Autodesk Fusion 360 part; units mm, degrees
(part 3 of 3)
equation "d13 = 1.525 mm + 0.5 mm"
named bodies: "PCB Motherboard", "Connection", "Top Layer", "Bottom Layer", "Connection (1)", "Connection (2)", "Connection (3)", "Connection (4)", "Connection (5)", "Connection (6)", "Connection (7)", "Connection (8)", "Connection (9)", "Connection (10)", "Connection (11)", "Connection (12)", "Connection (13)", "Connection (14)", "Top Layer (1)", "Top Layer (2)", "Top Layer (3)", "Top Layer (4)", "Top Layer (5)", "Top Layer (6)", "Top Layer (7)", "Top Layer (8)", "Top Layer (9)", "Top Layer (10)", "Top Layer (11)", "Top Layer (12)", "Top Layer (13)", "Top Layer (14)", "Bottom Layer (1)", "Bottom Layer (2)", "Bottom Layer (3)", "Bottom Layer (4)", "Bottom Layer (5)", "Bottom Layer (6)", "Bottom Layer (7)", "Bottom Layer (8)", "Bottom Layer (9)", "Bottom Layer (10)", "Bottom Layer (11)", "Bottom Layer (12)", "Bottom Layer (13)", "Bottom Layer (14)", "Connection (15)", "Connection (16)", "Connection (17)", "Connection (18)", "Connection (19)", "Connection (20)", "Connection (21)", "Connection (22)", "Connection (23)", "Connection (24)", "Connection (25)", "Connection (26)", "Connection (27)", "Connection (28)", "Connection (29)", "Connection (30)", "Connection (31)", "Connection (32)", "Connection (33)", "Connection (34)", "Connection (35)", "Connection (36)", "Connection (37)", "Connection (38)", "Connection (39)", "Connection (40)", "Connection (41)", "Connection (42)", "Connection (43)", "Connection (44)", "Connection (45)", "Connection (46)", "Connection (47)", "Connection (48)", "Connection (49)", "Connection (50)", "Connection (51)", "Connection (52)", "Connection (53)", "Connection (54)", "Connection (55)", "Connection (56)", "Connection (57)", "Connection (58)", "Connection (59)", "Connection (60)", "Connection (61)", "Connection (62)", "Connection (63)", "Connection (64)", "Connection (65)", "Connection (66)", "Connection (67)", "Connection (68)", "Connection (69)", "Connection (70)", "Connection (71)", "Connection (72)", "Connection (73)", "Connection (74)", "Connection (75)", "Connection (76)", "Connection (77)", "Connection (78)", "Connection (79)", "Connection (80)", "Connection (81)", "Connection (82)", "Connection (83)", "Connection (84)", "Connection (85)", "Connection (86)", "Connection (87)", "Connection (88)", "Connection (89)", "Connection (90)", "Connection (91)", "Connection (92)", "Connection (93)", "Connection (94)", "Connection (95)", "Connection (96)", "Connection (97)", "Connection (98)", "Connection (99)", "Connection (100)", "Connection (101)", "Connection (102)", "Connection (103)", "Connection (104)", "Connection (105)", "Connection (106)", "Connection (107)", "Connection (108)", "Connection (109)", "Connection (110)", "Connection (111)", "Connection (112)", "Connection (113)", "Connection (114)", "Connection (115)", "Connection (116)", "Connection (117)", "Connection (118)", "Connection (119)", "Connection (120)", "Connection (121)", "Connection (122)", "Connection (123)", "Connection (124)", "Connection (125)", "Connection (126)", "Connection (127)", "Connection (128)", "Connection (129)", "Connection (130)", "Connection (131)", "Connection (132)", "Connection (133)", "Connection (134)", "Connection (135)", "Connection (136)", "Connection (137)", "Connection (138)", "Connection (139)", "Connection (140)", "Connection (141)", "Connection (142)", "Connection (143)", "Connection (144)", "Connection (145)", "Connection (146)", "Connection (147)", "Connection (148)", "Connection (149)", "Connection (150)", "Connection (151)", "Connection (152)", "Connection (153)", "Connection (154)", "Connection (155)", "Connection (156)", "Connection (157)", "Connection (158)", "Connection (159)", "Connection (160)", "Connection (161)", "Connection (162)", "Connection (163)", "Connection (164)", "Connection (165)", "Connection (166)", "Connection (167)", "Connection (168)", "Connection (169)", "Connection (170)", "Connection (171)", "Connection (172)", "Connection (173)", "Connection (174)", "Connection (175)", "Connection (176)", "Connection (177)", "Connection (178)", "Connection (179)", "Connection (180)", "Connection (181)", "Connection (182)", "Connection (183)", "Connection (184)", "Connection (185)", "Connection (186)", "Connection (187)", "Connection (188)", "Connection (189)", "Connection (190)", "Connection (191)", "Connection (192)", "Connection (193)", "Connection (194)", "Connection (195)", "Connection (196)", "Connection (197)", "Connection (198)", "Connection (199)", "Connection (200)", "Connection (201)", "Connection (202)", "Connection (203)", "Connection (204)", "Connection (205)", "Connection (206)", "Connection (207)", "Connection (208)", "Connection (209)", "Connection (210)", "Connection (211)", "Connection (212)", "Connection (213)", "Connection (214)", "Connection (215)", "Connection (216)", "Connection (217)", "Connection (218)", "Connection (219)", "Connection (220)", "Connection (221)", "Connection (222)", "Connection (223)", "Connection (224)", "Connection (225)", "Connection (226)", "Connection (227)", "Connection (228)", "Connection (229)", "Connection (230)", "Connection (231)", "Connection (232)", "Connection (233)", "Connection (234)", "Connection (235)", "Connection (236)", "Connection (237)", "Connection (238)", "Connection (239)", "Connection (240)", "Connection (241)", "Connection (242)", "Connection (243)", "Connection (244)", "Connection (245)", "Connection (246)", "Connection (247)", "Connection (248)", "Connection (249)", "Connection (250)", "Connection (251)", "Connection (252)", "Connection (253)", "Connection (254)", "Connection (255)", "Connection (256)", "Connection (257)", "Connection (258)", "Connection (259)", "Connection (260)", "Connection (261)", "Connection (262)", "Connection (263)", "Connection (264)", "Connection (265)", "Connection (266)", "Connection (267)", "Connection (268)", "Connection (269)", "Connection (270)", "Connection (271)", "Connection (272)", "Connection (273)", "Connection (274)", "Connection (275)", "Connection (276)", "Connection (277)", "Connection (278)", "Connection (279)", "Connection (280)", "Connection (281)", "Connection (282)", "Connection (283)", "Connection (284)", "Connection (285)", "Connection (286)", "Connection (287)", "Connection (288)", "Connection (289)", "Connection (290)", "Connection (291)", "Connection (292)", "Connection (293)", "Connection (294)", "Connection (295)", "Connection (296)", "Connection (297)", "Connection (298)", "Connection (299)", "Connection (300)", "Connection (301)", "Connection (302)", "Connection (303)", "Connection (304)", "Connection (305)", "Connection (306)", "Connection (307)", "Connection (308)", "Connection (309)", "Connection (310)", "Connection (311)", "Connection (312)", "Connection (313)", "Connection (314)", "Connection (315)", "Connection (316)", "Connection (317)", "Connection (318)", "Connection (319)", "Connection (320)", "Connection (321)", "Connection (322)", "Connection (323)", "Connection (324)", "Connection (325)", "Connection (326)", "Connection (327)", "Connection (328)", "Connection (329)", "Connection (330)", "Connection (331)", "Connection (332)", "Connection (333)", "Connection (334)", "Connection (335)", "Connection (336)", "Connection (337)", "Connection (338)", "Connection (339)", "Connection (340)", "Connection (341)", "Connection (342)", "Connection (343)", "Connection (344)", "Connection (345)", "Connection (346)", "Connection (347)", "Connection (348)", "Connection (349)", "Connection (350)", "Connection (351)", "Connection (352)", "Connection (353)", "Connection (354)", "Connection (355)", "Connection (356)", "Connection (357)", "Connection (358)", "Connection (359)", "Connection (360)", "Connection (361)", "Connection (362)", "Connection (363)", "Connection (364)", "Connection (365)", "Connection (366)", "Connection (367)", "Connection (368)", "Connection (369)", "Connection (370)", "Connection (371)", "Connection (372)", "Connection (373)", "Connection (374)", "Top Layer (15)", "Top Layer (16)", "Top Layer (17)", "Top Layer (18)", "Top Layer (19)", "Top Layer (20)", "Top Layer (21)", "Top Layer (22)", "Top Layer (23)", "Top Layer (24)", "Top Layer (25)", "Top Layer (26)", "Top Layer (27)", "Top Layer (28)", "Top Layer (29)", "Top Layer (30)", "Top Layer (31)", "Top Layer (32)", "Top Layer (33)", "Top Layer (34)", "Top Layer (35)", "Top Layer (36)", "Top Layer (37)", "Top Layer (38)", "Top Layer (39)", "Top Layer (40)", "Top Layer (41)", "Top Layer (42)", "Top Layer (43)", "Top Layer (44)", "Top Layer (45)", "Top Layer (46)", "Top Layer (47)", "Top Layer (48)", "Top Layer (49)", "Top Layer (50)", "Top Layer (51)", "Top Layer (52)", "Top Layer (53)", "Top Layer (54)", "Top Layer (55)", "Top Layer (56)", "Top Layer (57)", "Top Layer (58)", "Top Layer (59)", "Top Layer (60)", "Top Layer (61)", "Top Layer (62)", "Top Layer (63)", "Top Layer (64)", "Top Layer (65)", "Top Layer (66)", "Top Layer (67)", "Top Layer (68)", "Top Layer (69)", "Top Layer (70)", "Top Layer (71)", "Top Layer (72)", "Top Layer (73)", "Top Layer (74)", "Top Layer (75)", "Top Layer (76)", "Top Layer (77)", "Top Layer (78)", "Top Layer (79)", "Top Layer (80)", "Top Layer (81)", "Top Layer (82)", "Top Layer (83)", "Top Layer (84)", "Top Layer (85)", "Top Layer (86)", "Top Layer (87)", "Top Layer (88)", "Top Layer (89)", "Top Layer (90)", "Top Layer (91)", "Top Layer (92)", "Top Layer (93)", "Top Layer (94)", "Top Layer (95)", "Top Layer (96)", "Top Layer (97)", "Top Layer (98)", "Top Layer (99)", "Top Layer (100)", "Top Layer (101)", "Top Layer (102)", "Top Layer (103)", "Top Layer (104)", "Top Layer (105)", "Top Layer (106)", "Top Layer (107)", "Top Layer (108)", "Top Layer (109)", "Top Layer (110)", "Top Layer (111)", "Top Layer (112)", "Top Layer (113)", "Top Layer (114)", "Top Layer (115)", "Top Layer (116)", "Top Layer (117)", "Top Layer (118)", "Top Layer (119)", "Top Layer (120)", "Top Layer (121)", "Top Layer (122)", "Top Layer (123)", "Top Layer (124)", "Top Layer (125)", "Top Layer (126)", "Top Layer (127)", "Top Layer (128)", "Top Layer (129)", "Top Layer (130)", "Top Layer (131)", "Top Layer (132)", "Top Layer (133)", "Top Layer (134)", "Top Layer (135)", "Top Layer (136)", "Top Layer (137)", "Top Layer (138)", "Top Layer (139)", "Top Layer (140)", "Top Layer (141)", "Top Layer (142)", "Top Layer (143)", "Top Layer (144)", "Top Layer (145)", "Top Layer (146)", "Top Layer (147)", "Top Layer (148)", "Top Layer (149)", "Top Layer (150)", "Top Layer (151)", "Top Layer (152)", "Top Layer (153)", "Top Layer (154)", "Top Layer (155)", "Top Layer (156)", "Top Layer (157)", "Top Layer (158)", "Top Layer (159)", "Top Layer (160)", "Top Layer (161)", "Top Layer (162)", "Top Layer (163)", "Top Layer (164)", "Top Layer (165)", "Top Layer (166)", "Top Layer (167)", "Top Layer (168)", "Top Layer (169)", "Top Layer (170)", "Top Layer (171)", "Top Layer (172)", "Top Layer (173)", "Top Layer (174)", "Top Layer (175)", "Top Layer (176)", "Top Layer (177)", "Top Layer (178)", "Top Layer (179)", "Top Layer (180)", "Top Layer (181)", "Top Layer (182)", "Top Layer (183)", "Top Layer (184)", "Top Layer (185)", "Top Layer (186)", "Top Layer (187)", "Top Layer (188)", "Top Layer (189)", "Top Layer (190)", "Top Layer (191)", "Top Layer (192)", "Top Layer (193)", "Top Layer (194)", "Top Layer (195)", "Top Layer (196)", "Top Layer (197)", "Top Layer (198)", "Top Layer (199)", "Top Layer (200)", "Top Layer (201)", "Top Layer (202)", "Top Layer (203)", "Top Layer (204)", "Top Layer (205)", "Top Layer (206)", "Top Layer (207)", "Top Layer (208)", "Top Layer (209)", "Top Layer (210)", "Top Layer (211)", "Top Layer (212)", "Top Layer (213)", "Top Layer (214)", "Top Layer (215)", "Top Layer (216)", "Top Layer (217)", "Top Layer (218)", "Top Layer (219)", "Top Layer (220)", "Top Layer (221)", "Top Layer (222)", "Top Layer (223)", "Top Layer (224)", "Top Layer (225)", "Top Layer (226)", "Top Layer (227)", "Top Layer (228)", "Top Layer (229)", "Top Layer (230)", "Top Layer (231)", "Top Layer (232)", "Top Layer (233)", "Top Layer (234)", "Top Layer (235)", "Top Layer (236)", "Top Layer (237)", "Top Layer (238)", "Top Layer (239)", "Top Layer (240)", "Top Layer (241)", "Top Layer (242)", "Top Layer (243)", "Top Layer (244)", "Top Layer (245)", "Top Layer (246)", "Top Layer (247)", "Top Layer (248)", "Top Layer (249)", "Top Layer (250)", "Top Layer (251)", "Top Layer (252)", "Top Layer (253)", "Top Layer (254)", "Top Layer (255)", "Top Layer (256)", "Top Layer (257)", "Top Layer (258)", "Top Layer (259)", "Top Layer (260)", "Top Layer (261)", "Top Layer (262)", "Top Layer (263)", "Top Layer (264)", "Top Layer (265)", "Top Layer (266)", "Top Layer (267)", "Top Layer (268)", "Top Layer (269)", "Top Layer (270)", "Top Layer (271)", "Top Layer (272)", "Top Layer (273)", "Top Layer (274)", "Top Layer (275)", "Top Layer (276)", "Top Layer (277)", "Top Layer (278)", "Top Layer (279)", "Top Layer (280)", "Top Layer (281)", "Top Layer (282)", "Top Layer (283)", "Top Layer (284)", "Top Layer (285)", "Top Layer (286)", "Top Layer (287)", "Top Layer (288)", "Top Layer (289)", "Top Layer (290)", "Top Layer (291)", "Top Layer (292)", "Top Layer (293)", "Top Layer (294)", "Top Layer (295)", "Top Layer (296)", "Top Layer (297)", "Top Layer (298)", "Top Layer (299)", "Top Layer (300)", "Top Layer (301)", "Top Layer (302)", "Top Layer (303)", "Top Layer (304)", "Top Layer (305)", "Top Layer (306)", "Top Layer (307)", "Top Layer (308)", "Top Layer (309)", "Top Layer (310)", "Top Layer (311)", "Top Layer (312)", "Top Layer (313)", "Top Layer (314)", "Top Layer (315)", "Top Layer (316)", "Top Layer (317)", "Top Layer (318)", "Top Layer (319)", "Top Layer (320)", "Top Layer (321)", "Top Layer (322)", "Top Layer (323)", "Top Layer (324)", "Top Layer (325)", "Top Layer (326)", "Top Layer (327)", "Top Layer (328)", "Top Layer (329)", "Top Layer (330)", "Top Layer (331)", "Top Layer (332)", "Top Layer (333)", "Top Layer (334)", "Top Layer (335)", "Top Layer (336)", "Top Layer (337)", "Top Layer (338)", "Top Layer (339)", "Top Layer (340)", "Top Layer (341)", "Top Layer (342)", "Top Layer (343)", "Top Layer (344)", "Top Layer (345)", "Top Layer (346)", "Top Layer (347)", "Top Layer (348)", "Top Layer (349)", "Top Layer (350)", "Top Layer (351)", "Top Layer (352)", "Top Layer (353)", "Top Layer (354)", "Top Layer (355)", "Top Layer (356)", "Top Layer (357)", "Top Layer (358)", "Top Layer (359)", "Top Layer (360)", "Top Layer (361)", "Top Layer (362)", "Top Layer (363)", "Top Layer (364)", "Top Layer (365)", "Top Layer (366)", "Top Layer (367)", "Top Layer (368)", "Top Layer (369)", "Top Layer (370)", "Top Layer (371)", "Top Layer (372)", "Top Layer (373)", "Top Layer (374)", "Bottom Layer (15)", "Bottom Layer (16)", "Bottom Layer (17)", "Bottom Layer (18)", "Bottom Layer (19)", "Bottom Layer (20)", "Bottom Layer (21)", "Bottom Layer (22)", "Bottom Layer (23)", "Bottom Layer (24)", "Bottom Layer (25)", "Bottom Layer (26)", "Bottom Layer (27)", "Bottom Layer (28)", "Bottom Layer (29)", "Bottom Layer (30)", "Bottom Layer (31)", "Bottom Layer (32)", "Bottom Layer (33)", "Bottom Layer (34)", "Bottom Layer (35)", "Bottom Layer (36)", "Bottom Layer (37)", "Bottom Layer (38)", "Bottom Layer (39)", "Bottom Layer (40)", "Bottom Layer (41)", "Bottom Layer (42)", "Bottom Layer (43)", "Bottom Layer (44)", "Bottom Layer (45)", "Bottom Layer (46)", "Bottom Layer (47)", "Bottom Layer (48)", "Bottom Layer (49)", "Bottom Layer (50)", "Bottom Layer (51)", "Bottom Layer (52)", "Bottom Layer (53)", "Bottom Layer (54)", "Bottom Layer (55)", "Bottom Layer (56)", "Bottom Layer (57)", "Bottom Layer (58)", "Bottom Layer (59)", "Bottom Layer (60)", "Bottom Layer (61)", "Bottom Layer (62)", "Bottom Layer (63)", "Bottom Layer (64)", "Bottom Layer (65)", "Bottom Layer (66)", "Bottom Layer (67)", "Bottom Layer (68)", "Bottom Layer (69)", "Bottom Layer (70)", "Bottom Layer (71)", "Bottom Layer (72)", "Bottom Layer (73)", "Bottom Layer (74)", "Bottom Layer (75)", "Bottom Layer (76)", "Bottom Layer (77)", "Bottom Layer (78)", "Bottom Layer (79)", "Bottom Layer (80)", "Bottom Layer (81)", "Bottom Layer (82)", "Bottom Layer (83)", "Bottom Layer (84)", "Bottom Layer (85)", "Bottom Layer (86)", "Bottom Layer (87)", "Bottom Layer (88)", "Bottom Layer (89)", "Bottom Layer (90)", "Bottom Layer (91)", "Bottom Layer (92)", "Bottom Layer (93)", "Bottom Layer (94)", "Bottom Layer (95)", "Bottom Layer (96)", "Bottom Layer (97)", "Bottom Layer (98)", "Bottom Layer (99)", "Bottom Layer (100)", "Bottom Layer (101)", "Bottom Layer (102)", "Bottom Layer (103)", "Bottom Layer (104)", "Bottom Layer (105)", "Bottom Layer (106)", "Bottom Layer (107)", "Bottom Layer (108)", "Bottom Layer (109)", "Bottom Layer (110)", "Bottom Layer (111)", "Bottom Layer (112)", "Bottom Layer (113)", "Bottom Layer (114)", "Bottom Layer (115)", "Bottom Layer (116)", "Bottom Layer (117)", "Bottom Layer (118)", "Bottom Layer (119)", "Bottom Layer (120)", "Bottom Layer (121)", "Bottom Layer (122)", "Bottom Layer (123)", "Bottom Layer (124)", "Bottom Layer (125)", "Bottom Layer (126)", "Bottom Layer (127)", "Bottom Layer (128)", "Bottom Layer (129)", "Bottom Layer (130)", "Bottom Layer (131)", "Bottom Layer (132)", "Bottom Layer (133)", "Bottom Layer (134)", "Bottom Layer (135)", "Bottom Layer (136)", "Bottom Layer (137)", "Bottom Layer (138)", "Bottom Layer (139)", "Bottom Layer (140)", "Bottom Layer (141)", "Bottom Layer (142)", "Bottom Layer (143)", "Bottom Layer (144)", "Bottom Layer (145)", "Bottom Layer (146)", "Bottom Layer (147)", "Bottom Layer (148)", "Bottom Layer (149)", "Bottom Layer (150)", "Bottom Layer (151)", "Bottom Layer (152)", "Bottom Layer (153)", "Bottom Layer (154)", "Bottom Layer (155)", "Bottom Layer (156)", "Bottom Layer (157)", "Bottom Layer (158)", "Bottom Layer (159)", "Bottom Layer (160)", "Bottom Layer (161)", "Bottom Layer (162)", "Bottom Layer (163)", "Bottom Layer (164)", "Bottom Layer (165)", "Bottom Layer (166)", "Bottom Layer (167)", "Bottom Layer (168)", "Bottom Layer (169)", "Bottom Layer (170)", "Bottom Layer (171)", "Bottom Layer (172)", "Bottom Layer (173)", "Bottom Layer (174)", "Bottom Layer (175)", "Bottom Layer (176)", "Bottom Layer (177)", "Bottom Layer (178)", "Bottom Layer (179)", "Bottom Layer (180)", "Bottom Layer (181)", "Bottom Layer (182)", "Bottom Layer (183)", "Bottom Layer (184)", "Bottom Layer (185)", "Bottom Layer (186)", "Bottom Layer (187)", "Bottom Layer (188)", "Bottom Layer (189)", "Bottom Layer (190)", "Bottom Layer (191)", "Bottom Layer (192)", "Bottom Layer (193)", "Bottom Layer (194)", "Bottom Layer (195)", "Bottom Layer (196)", "Bottom Layer (197)", "Bottom Layer (198)", "Bottom Layer (199)", "Bottom Layer (200)", "Bottom Layer (201)", "Bottom Layer (202)", "Bottom Layer (203)", "Bottom Layer (204)", "Bottom Layer (205)", "Bottom Layer (206)", "Bottom Layer (207)", "Bottom Layer (208)", "Bottom Layer (209)", "Bottom Layer (210)", "Bottom Layer (211)", "Bottom Layer (212)", "Bottom Layer (213)", "Bottom Layer (214)", "Bottom Layer (215)", "Bottom Layer (216)", "Bottom Layer (217)", "Bottom Layer (218)", "Bottom Layer (219)", "Bottom Layer (220)", "Bottom Layer (221)", "Bottom Layer (222)", "Bottom Layer (223)", "Bottom Layer (224)", "Bottom Layer (225)", "Bottom Layer (226)", "Bottom Layer (227)", "Bottom Layer (228)", "Bottom Layer (229)", "Bottom Layer (230)", "Bottom Layer (231)", "Bottom Layer (232)", "Bottom Layer (233)", "Bottom Layer (234)", "Bottom Layer (235)", "Bottom Layer (236)", "Bottom Layer (237)", "Bottom Layer (238)", "Bottom Layer (239)", "Bottom Layer (240)", "Bottom Layer (241)", "Bottom Layer (242)", "Bottom Layer (243)", "Bottom Layer (244)", "Bottom Layer (245)", "Bottom Layer (246)", "Bottom Layer (247)", "Bottom Layer (248)", "Bottom Layer (249)", "Bottom Layer (250)", "Bottom Layer (251)", "Bottom Layer (252)", "Bottom Layer (253)", "Bottom Layer (254)", "Bottom Layer (255)", "Bottom Layer (256)", "Bottom Layer (257)", "Bottom Layer (258)", "Bottom Layer (259)", "Bottom Layer (260)", "Bottom Layer (261)", "Bottom Layer (262)", "Bottom Layer (263)", "Bottom Layer (264)", "Bottom Layer (265)", "Bottom Layer (266)", "Bottom Layer (267)", "Bottom Layer (268)", "Bottom Layer (269)", "Bottom Layer (270)", "Bottom Layer (271)", "Bottom Layer (272)", "Bottom Layer (273)", "Bottom Layer (274)", "Bottom Layer (275)", "Bottom Layer (276)", "Bottom Layer (277)", "Bottom Layer (278)", "Bottom Layer (279)", "Bottom Layer (280)", "Bottom Layer (281)", "Bottom Layer (282)", "Bottom Layer (283)", "Bottom Layer (284)", "Bottom Layer (285)", "Bottom Layer (286)", "Bottom Layer (287)", "Bottom Layer (288)", "Bottom Layer (289)", "Bottom Layer (290)", "Bottom Layer (291)", "Bottom Layer (292)", "Bottom Layer (293)", "Bottom Layer (294)", "Bottom Layer (295)", "Bottom Layer (296)", "Bottom Layer (297)", "Bottom Layer (298)", "Bottom Layer (299)", "Bottom Layer (300)", "Bottom Layer (301)", "Bottom Layer (302)", "Bottom Layer (303)", "Bottom Layer (304)", "Bottom Layer (305)", "Bottom Layer (306)", "Bottom Layer (307)", "Bottom Layer (308)", "Bottom Layer (309)", "Bottom Layer (310)", "Bottom Layer (311)", "Bottom Layer (312)", "Bottom Layer (313)", "Bottom Layer (314)", "Bottom Layer (315)", "Bottom Layer (316)", "Bottom Layer (317)", "Bottom Layer (318)", "Bottom Layer (319)", "Bottom Layer (320)", "Bottom Layer (321)", "Bottom Layer (322)", "Bottom Layer (323)", "Bottom Layer (324)", "Bottom Layer (325)", "Bottom Layer (326)", "Bottom Layer (327)", "Bottom Layer (328)", "Bottom Layer (329)", "Bottom Layer (330)", "Bottom Layer (331)", "Bottom Layer (332)", "Bottom Layer (333)", "Bottom Layer (334)", "Bottom Layer (335)", "Bottom Layer (336)", "Bottom Layer (337)", "Bottom Layer (338)", "Bottom Layer (339)", "Bottom Layer (340)", "Bottom Layer (341)", "Bottom Layer (342)", "Bottom Layer (343)", "Bottom Layer (344)", "Bottom Layer (345)", "Bottom Layer (346)", "Bottom Layer (347)", "Bottom Layer (348)", "Bottom Layer (349)", "Bottom Layer (350)", "Bottom Layer (351)", "Bottom Layer (352)", "Bottom Layer (353)", "Bottom Layer (354)", "Bottom Layer (355)", "Bottom Layer (356)", "Bottom Layer (357)", "Bottom Layer (358)", "Bottom Layer (359)", "Bottom Layer (360)", "Bottom Layer (361)", "Bottom Layer (362)", "Bottom Layer (363)", "Bottom Layer (364)", "Bottom Layer (365)", "Bottom Layer (366)", "Bottom Layer (367)", "Bottom Layer (368)", "Bottom Layer (369)", "Bottom Layer (370)", "Bottom Layer (371)", "Bottom Layer (372)", "Bottom Layer (373)", "Bottom Layer (374)"
